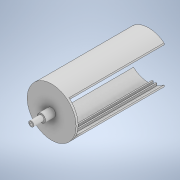
# Autodesk Inventor part: Casing
Saved by Autodesk Inventor 2020 (Build 240168000, 168)
## iProperties
Created: 2021-06-18
Part Number: Casing
Material: Generic
Document SubType Name: Modeling
Designer: ugwue
Density: 1 g/cm^3
Appearance: Default
Author: ugwue
Autodesk Inventor part; units mm, degrees
ref_plane "YZ Plane" through (0, 0, 0) normal (1, 0, 0) x (0, 1, 0)
ref_plane "XZ Plane" through (0, 0, 0) normal (0, 1, 0) x (-1, 0, 0)
ref_plane "XY Plane" through (0, 0, 0) normal (0, 0, 1) x (1, 0, 0)
sketch "Sketch1" plane through (0, 0, 0) normal (0, 0, 1) x (1, 0, 0)
  circle A0 centre (10, 32.5) radius 36
  line L0 (22, 0.6881) -> (22, 4)
  line L1 (22, 4) -> (20, 4)
  line L2 (20, 4) -> (20, 0)
  line L3 (16.7, 4) -> (15, 4)
  line L4 (22, 64.3119) -> (22, 61)
  line L5 (22, 61) -> (20, 61)
  line L6 (20, 61) -> (20, 65)
  line L7 (16.7, 61) -> (15, 61)
  line L8 (16.7, 61) -> (14.7, 61)
  line L9 (14.7, 61) -> (14.7, 66.1736)
  line L10 (16.7, 65.8333) -> (16.7, 61)
  line L11 (16.7, 4) -> (14.7, 4)
  line L12 (14.7, 4) -> (14.7, -1.1736)
  line L13 (16.7, -0.8333) -> (16.7, 4)
  arc A1 (16.7, -0.8333) -> (20, 0.0038) centre (10, 32.5) ccw
  arc A2 (14.7, 66.1736) -> (14.7, -1.1736) centre (10, 32.5) ccw
  arc A3 (22, 0.6881) -> (22, 64.3119) centre (10, 32.5) ccw
  arc A4 (20, 64.9962) -> (16.7, 65.8333) centre (10, 32.5) ccw
  point P0 (0, 0)
  constraints: 28 end point, 8 point on circle, 5 centre point, 4 horizontal, 4 parallel, 3 point on line, 2 perpendicular, 1 coincident
extrude "Extrusion1" add sketch "Sketch1" along normal blind 140
sketch "Sketch2" plane through (10, 32.5, 140) normal (0, 0, 1) x (1, 0, 0)
  circle A0 centre (0, 0) radius 36
  point P0 (-10, -32.5)
  constraints: 1 centre point
extrude "Extrusion2" add sketch "Sketch2" along normal blind 3
sketch "Sketch3" plane through (10, 32.5, 143) normal (0, 0, 1) x (1, 0, 0)
  circle A0 centre (0, 0) radius 3.85
  arc A1 (-2.15, -1.2757) -> (-2.15, 1.2757) centre (0, 0) ccw
  line L0 (-2.15, 0) -> (-2.15, 1.2757)
  line L1 (-2.15, 0) -> (-2.15, -1.2757)
  point P0 (-10, -32.5)
  dimension "d14" = 7.7
  dimension "d15" = 5
  constraints: 4 end point, 2 centre point, 2 point on circle, 1 coincident, 1 point on line
  measures "d14" diameter of A0
  measures "d15" diameter of A1
extrude "Extrusion3" add sketch "Sketch3" along normal blind 30
sketch "Sketch4" plane through (10, 32.5, 143) normal (0, 0, 1) x (1, 0, 0)
  circle A0 centre (0, 0) radius 6
  point P0 (-10, -32.5)
  dimension "d19" = 12
  constraints: 1 centre point
  measures "d19" diameter of A0
extrude "Extrusion4" add sketch "Sketch4" along normal blind 15
sketch "Sketch5" plane through (10, 32.5, 0) normal (0, 0, -1) x (-1, 0, 0)
  line L0 (-22.5, 36.2326) -> (-22.5, -36.2326)
  line L1 (-22.5, -36.2326) -> (22.5, -36.2326)
  line L2 (22.5, -36.2326) -> (22.5, 36.2326)
  line L3 (22.5, 36.2326) -> (-22.5, 36.2326)
  line L4 (-22.5, 36.2326) -> (22.5, -36.2326) construction
  line L5 (-22.5, -36.2326) -> (22.5, 36.2326) construction
  circle A0 centre (0, 0) radius 36
  point P0 (10, -32.5)
  point P1 (-22.5, -28.1025)
  point P2 (-22.5, 28.1025)
  point P3 (22.5, 28.1025)
  point P4 (22.5, -28.1025)
  dimension "d22" = 45
  dimension "d25" = 72.4652
  constraints: 12 end point, 2 midpoint, 2 parallel, 1 centre point, 1 coincident, 1 perpendicular, 1 vertical
  measures "d22" distance of L1.end L0.end
  measures "d25" distance of L0.start L0.end
extrude "Extrusion5" cut sketch "Sketch5" against normal blind 140 contours L0 A0 | A0 L2
body "Solid1"
